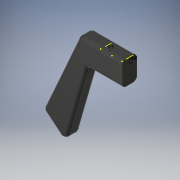
# Autodesk Inventor part: Handle Gearbox handle
Saved by Autodesk Inventor 2018 (Build 220112000, 112)
## iProperties
Created: 2017-08-08
Part Number: Handle Gearbox handle
Material: ABS Plastic
Document SubType Name: Modeling
Designer: M227562
Density: 1.06 g/cm^3
Appearance: Smooth - Black
Author: M227562
Autodesk Inventor part; units mm, degrees
ref_plane "YZ Plane" through (0, 0, 0) normal (1, 0, 0) x (0, 1, 0)
ref_plane "XZ Plane" through (0, 0, 0) normal (0, 1, 0) x (-1, 0, 0)
ref_plane "XY Plane" through (0, 0, 0) normal (0, 0, 1) x (1, 0, 0)
sketch "Sketch4" plane through (0, 0, 0) normal (0, 1, 0) x (-1, 0, 0)
  line L0 (23.5565, -2.3733) -> (57.8608, -79.438)
  line L1 (0, 0) -> (0, -24)
  line L2 (0, -24) -> (11.8861, -24)
  line L3 (56.7451, -84.1558) -> (41.5484, -96.6361)
  line L4 (35.1649, -94.6478) -> (15.731, -26.8971)
  line L5 (19.9022, 0) -> (0, 0)
  arc A0 (15.731, -26.8971) -> (11.8861, -24) centre (11.8861, -28) ccw
  arc A1 (23.5565, -2.3733) -> (19.9022, 0) centre (19.9022, -4) ccw
  arc A2 (56.7451, -84.1558) -> (57.8608, -79.438) centre (54.2065, -81.0647) ccw
  arc A3 (35.1649, -94.6478) -> (41.5484, -96.6361) centre (39.0098, -93.5449) ccw
  point P0 (22.5, 0)
  point P1 (59.1, -82.2219)
  point P2 (36.8435, -100.5)
  dimension "d40" = 22.5
  dimension "d41" = 90
  dimension "d43" = 24
  dimension "d44" = 28.8
  dimension "d45" = 4
  constraints: 12 end point, 8 point on circle, 8 tangent, 6 point on line, 4 centre point, 3 equal radius, 1 perpendicular
  measures "d40" distance of L1.start point (22.5, 0)
  measures "d41" distance of point (22.5, 0) point (59.1, -82.222)
  measures "d43" distance of L1.start L1.end
  measures "d44" distance of point (59.1, -82.222) point (36.844, -100.5)
  measures "d45" radius of A0
extrude "Extrusion3" add sketch "Sketch4" along normal blind 15
fillet "Fillet3" radius 4 18 edges at (-37.8203, 15, -97.364) (-49.1468, 15, -90.396) (-58.0991, 15, -81.9852) (-40.7086, 15, -40.9057) (-22.0808, 15, -0.6454) (-9.9511, 15, 0) (-14.2932, 15, -24.8053) (-5.943, 15, -24) (-25.4479, 15, -60.7725) (-37.8203, 0, -97.364) (-49.1468, 0, -90.396) (-58.0991, 0, -81.9852) (-40.7086, 0, -40.9057) (-22.0808, 0, -0.6454) (-9.9511, 0, 0) (-14.2932, 0, -24.8053) (-5.943, 0, -24) (-25.4479, 0, -60.7725)
sketch "Sketch5" plane through (0, 0, -4) normal (1, 0, 0) x (0, 0, -1)
  line L0 (-4, 4) -> (-4, 11) projected
  line L1 (-4, 7.5) -> (1.9, 7.5)
  point P0 (-4, 0)
  dimension "d49" = 5.9
  constraints: 2 end point, 1 horizontal, 1 midpoint
  measures "d49" distance of L1.start L1.end
sketch "Sketch6" plane through (0, 0, -4) normal (1, 0, 0) x (0, 0, -1)
  line L0 (0, 0) -> (16, 0) projected
  line L1 (20, 4) -> (20, 11) projected
  arc A0 (16, 0) -> (20, 4) centre (16, 4) ccw
  arc A1 (-4, 4) -> (0, 0) centre (0, 4) ccw projected
  arc A2 (0, 15) -> (-4, 11) centre (0, 11) ccw projected
  arc A3 (0, 15) -> (0, 15) centre (0, 11) ccw
  arc A4 (20, 11) -> (16, 15) centre (16, 11) ccw projected
  line L2 (16, 15) -> (0, 15)
  line L3 (-4, 4) -> (-4, 11) projected
  line L4 (-4, 11) -> (-4, 4)
  arc A5 (0, 15) -> (-4, 11) centre (0, 11) ccw projected
  point P0 (-4, 0)
  constraints: 4 end point, 3 point on circle, 1 centre point, 1 collinear, 1 horizontal, 1 tangent, 1 vertical alignment, 3 other
extrude "Extrusion4" add sketch "Sketch6" along normal blind 11.5
sketch "Sketch7" plane through (11.5, 0, -4) normal (1, 0, 0) x (0, 0, -1)
  point P0 (-4, 0)
sketch "Sketch8" plane through (11.5, 0, -4) normal (1, 0, 0) x (0, 0, -1)
  line L0 (-4, 4) -> (-4, 11) projected
  arc A0 (16, 0) -> (20, 4) centre (16, 4) ccw projected
  line L1 (20, 4) -> (20, 11) projected
  line L2 (20, 4) -> (20, 11)
  line L3 (77.0647, 0) -> (0, 0) projected
  arc A1 (-4, 4) -> (0, 0) centre (0, 4) ccw projected
  line L4 (16, 0) -> (0, 0)
  arc A2 (20, 11) -> (16, 15) centre (16, 11) ccw projected
  line L5 (0, 15) -> (77.0647, 15) projected
  line L6 (16, 15) -> (0, 15)
  arc A3 (20, 11) -> (16, 15) centre (16, 11) ccw
  arc A4 (16, 0.4098) -> (20, 4) centre (16.6189, 3.7436) ccw
  arc A5 (-4, 4) -> (0, 0) centre (0, 4) ccw
  ellipse E0 centre (0, 11) end of major axis (0, 15) minor radius 1.6267 (0, 15) -> (-1.6267, 11) ccw projected
  arc A6 (0, 15) -> (-4, 11) centre (0, 11) ccw
  point P0 (-4, 0)
  constraints: 9 point on circle, 6 end point, 6 tangent, 4 centre point, 2 collinear, 2 point on line, 1 concentric, 1 horizontal, 2 other
extrude "Extrusion5" add sketch "Sketch8" along normal blind 10 contours L0 A6 L5 A2 L1 A0 L3 A1
sketch "Sketch9" plane through (21.5, 0, -4) normal (1, 0, 0) x (0, 0, -1)
  line L0 (-4, 4) -> (-4, 11) projected
  line L1 (-4, 7.5) -> (1.9, 7.5)
  point P0 (-4, 0)
  dimension "d56" = 5.9
  constraints: 2 end point, 1 horizontal, 1 midpoint
  measures "d56" distance of L1.start L1.end
sketch "Sketch10" plane through (21.5, 0, -4) normal (1, 0, 0) x (0, 0, -1)
  line L0 (-4, 4) -> (-4, 11) projected
  line L1 (-4, 7.5) -> (1.9, 7.5)
  point P0 (-4, 0)
  dimension "d57" = 5.9
  constraints: 2 end point, 1 horizontal, 1 midpoint
  measures "d57" distance of L1.start L1.end
body "Solid3"
